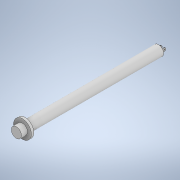
# Autodesk Inventor part: 顶杆
Saved by Autodesk Inventor 2022 (Build 260153000, 153)
## iProperties
Created: 2023-02-22
Part Number: 顶杆
Material: 常规
Document SubType Name: Modeling
Designer: 李承轩
Density: 1 g/cm^3
Appearance: 默认
Author: 李承轩
Autodesk Inventor part; units mm, degrees
ref_plane "YZ Plane" through (0, 0, 0) normal (1, 0, 0) x (0, 1, 0)
ref_plane "XZ Plane" through (0, 0, 0) normal (0, 1, 0) x (-1, 0, 0)
ref_plane "XY Plane" through (0, 0, 0) normal (0, 0, 1) x (1, 0, 0)
sketch "草图1" plane through (0, 0, 0) normal (0, 0, 1) x (1, 0, 0)
  circle A0 centre (0, 0) radius 10
  dimension "d0" = 20
  constraints: 1 centre point, 1 coincident
  measures "d0" diameter of A0
extrude "拉伸1" add sketch "草图1" along normal mid plane 280
sketch "草图2" plane through (0, 0, -140) normal (0, 0, -1) x (-1, 0, 0)
  line L0 (-4.5, 3) -> (-3, 3)
  line L1 (-3, 3) -> (-3, -3)
  line L2 (-3, -3) -> (-4.5, -3)
  line L3 (-4.5, -3) -> (-4.5, 3)
  line L4 (0, 0) -> (0, 6.2448)
  line L5 (4.5, 3) -> (3, 3)
  line L6 (3, 3) -> (3, -3)
  line L7 (3, -3) -> (4.5, -3)
  line L8 (4.5, -3) -> (4.5, 3)
  point P0 (-3, 0)
  point P1 (3, 0)
  dimension "d3" = 1.5
  dimension "d4" = 6
  dimension "d5" = 6
  constraints: 18 end point, 5 symmetric about line, 2 parallel, 1 horizontal, 1 horizontal alignment, 1 midpoint, 1 perpendicular, 1 vertical
  measures "d3" distance of L1.end L2.end
  measures "d4" distance of L0.end L1.end
  measures "d5" distance of point (3, 0) point (-3, 0)
extrude "拉伸2" add sketch "草图2" along normal blind 10
full round fillet "全圆角1" first side at (4, -3, -143.3333) centre faces at (4, 1, -150) second side at (3.5, 3, -143.3333)
full round fillet "全圆角2" first side at (-3.5, -3, -143.3333) centre faces at (-3.5, 1, -150) second side at (-4, 3, -143.3333)
sketch "草图3" plane through (-4.5, -3, -140) normal (-1, 0, 0) x (0, 0, 1)
  arc A0 (-7, 6) -> (-7, 0) centre (-7, 3) ccw projected
  point P0 (140, 3)
  constraints: 1 coincident
hole "孔1" at (-4.5, 0, -147) direction (1, 0, 0) diameter 2 end through all
ref_plane "工作平面1" through (0, 0, 123) normal (0, 0, 1) x (1, 0, 0)
sketch "草图4" plane through (0, 0, 123) normal (0, 0, 1) x (1, 0, 0)
  circle A0 centre (0, 0) radius 17.5
  dimension "d16" = 35
  constraints: 1 centre point, 1 coincident
  measures "d16" diameter of A0
extrude "拉伸3" add sketch "草图4" along normal blind 5
